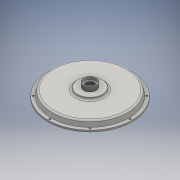
# Autodesk Inventor part: Flasque 1
Saved by Autodesk Inventor 2016 (Build 200138000, 138)
## iProperties
Created: 2015-11-14
Part Number: Flasque 1
Material: Générique
Document SubType Name: Modeling
Designer: Cyril
Density: 1 g/cm^3
Appearance: Par défaut
Author: Cyril
Autodesk Inventor part; units mm, degrees
ref_plane "YZ Plane" through (0, 0, 0) normal (1, 0, 0) x (0, 1, 0)
ref_plane "XZ Plane" through (0, 0, 0) normal (0, 1, 0) x (-1, 0, 0)
ref_plane "XY Plane" through (0, 0, 0) normal (0, 0, 1) x (1, 0, 0)
sketch "Esquisse1" plane through (0, 0, 0) normal (1, 0, 0) x (0, 1, 0)
  line L0 (0, 0) -> (0, 42.75) construction
  line L1 (102.5, -2.5) -> (106.5, -2.5)
  line L2 (106.5, -2.5) -> (106.5, 0)
  line L3 (106.5, 0) -> (115, 0)
  line L4 (115, 0) -> (115, 4.6)
  line L5 (115, 4.6) -> (106, 4.6)
  line L6 (106, 4.6) -> (103.0675, 15.5441)
  arc A0 (103.0675, 15.5441) -> (98.2379, 19.25) centre (98.2379, 14.25) ccw
  line L7 (98.2379, 19.25) -> (40, 19.25)
  line L8 (15, 39.25) -> (16.5, 39.25)
  line L9 (16.5, 39.25) -> (17.5, 38.25)
  line L10 (17.5, 38.25) -> (17.5, 27.25)
  line L11 (17.5, 27.25) -> (16.5, 27.25)
  line L12 (16.5, 27.25) -> (16.5, 25.25)
  line L13 (16.5, 25.25) -> (34, 25.25)
  line L14 (34, 25.25) -> (35, 24.25)
  arc A1 (35, 24.25) -> (40, 19.25) centre (40, 24.25) ccw
  line L15 (98.6398, 14.75) -> (34.5, 14.75)
  line L16 (102.3296, 6.7069) -> (100.5717, 13.2676)
  arc A2 (100.5717, 13.2676) -> (98.6398, 14.75) centre (98.6398, 12.75) ccw
  line L17 (102.5, -2.5) -> (102.5, 5.4128)
  arc A3 (102.5, 5.4128) -> (102.3296, 6.7069) centre (97.5, 5.4128) ccw
  line L18 (29.5, 9.75) -> (29.5, 8.25)
  arc A4 (34.5, 14.75) -> (29.5, 9.75) centre (34.5, 9.75) ccw
  line L19 (29.5, 8.25) -> (22, 8.25)
  line L20 (22, 8.25) -> (22, 20.25)
  line L21 (22, 20.25) -> (18.5, 20.25)
  line L22 (18.5, 20.25) -> (18.5, 21.25)
  line L23 (18.5, 21.25) -> (11.7, 26.95)
  line L24 (11.7, 26.95) -> (11.7, 32.25)
  line L25 (11.7, 32.25) -> (15, 32.25)
  line L26 (15, 32.25) -> (15, 39.25)
  line L27 (40, 24.25) -> (35, 24.25) construction
  dimension "d0" = 115
  dimension "d1" = 106.5
  dimension "d3" = 2.5
  dimension "d4" = 4.6
  dimension "d5" = 0.5
  dimension "d8" = 5
  dimension "d16" = 105
  dimension "d17" = 42.75
  dimension "d40" = 39.25
  dimension "d42" = 1
  dimension "d43" = 1
  dimension "d45" = 1
  dimension "d46" = 2
  dimension "d47" = 1
  dimension "d48" = 1
  dimension "d49" = 5
  dimension "d50" = 17.5
  dimension "d51" = 35
  dimension "d56" = 23.5
  dimension "d57" = 3
  dimension "d58" = 4.5
  dimension "d59" = 2
  dimension "d60" = 102.5
  dimension "d61" = 5
  dimension "d62" = 5
  dimension "d63" = 22
  dimension "d64" = 29.5
  dimension "d65" = 17
  dimension "d66" = 12
  dimension "d67" = 18.5
  dimension "d68" = 1
  dimension "d69" = 5.7
  dimension "d70" = 6.8
  dimension "d71" = 7
  dimension "d72" = 15
  constraints: 56 end point, 10 horizontal, 10 point on circle, 9 tangent, 8 vertical, 5 centre point, 5 perpendicular, 3 point on line, 1 parallel
  measures "d0" distance between parallel lines of L0 L4
  measures "d1" distance between parallel lines of L0 L2
  measures "d3" distance of L1.end L2.end
  measures "d4" distance of L3.end L4.end
  measures "d5" distance from line of L2 L5.end
  measures "d8" radius of A0
  measures "d16" angle of L5 L6
  measures "d17" distance of L0.start L0.end
  measures "d40" distance between parallel lines of L3 L8
  measures "d42" horizontal distance of L8.end L9.end
  measures "d43" horizontal distance of L8.end L9.end
  measures "d45" distance of L10.end L11.end
  measures "d46" distance of L11.end L12.end
  measures "d47" horizontal distance of L13.end L14.end
  measures "d48" horizontal distance of L13.end L14.end
  measures "d49" radius of A1
  measures "d50" distance between parallel lines of L0 L10
  measures "d51" distance from line of L0 L14.end
  measures "d56" distance from line of L7 L0.end
  measures "d57" distance between parallel lines of L16 L6
  measures "d58" distance between parallel lines of L7 L15
  measures "d59" radius of A2
  measures "d60" distance between parallel lines of L0 L17
  measures "d61" radius of A3
  measures "d62" radius of A4
  measures "d63" distance between parallel lines of L0 L20
  measures "d64" distance between parallel lines of L0 L18
  measures "d65" distance between parallel lines of L13 L19
  measures "d66" distance of L19.end L20.end
  measures "d67" distance between parallel lines of L0 L22
  measures "d68" distance of L21.end L22.end
  measures "d69" vertical distance of L22.end L23.end
  measures "d70" horizontal distance of L22.end L23.end
  measures "d71" distance of L25.end L8.start
  measures "d72" distance between parallel lines of L0 L26
revolve "Révolution1" add sketch "Esquisse1" angle 360 about axis through (0, 0, 0) along (0, 0, 1)
sketch "Esquisse2" plane through (0, 0, 4.6) normal (0, 0, 1) x (1, 0, 0)
  circle A0 centre (-110, 0) radius 2.65
  circle A1 centre (-77.7817, 77.7817) radius 2.65
  circle A2 centre (0, 110) radius 2.65
  circle A3 centre (77.7817, 77.7817) radius 2.65
  circle A4 centre (110, 0) radius 2.65
  circle A5 centre (77.7817, -77.7817) radius 2.65
  circle A6 centre (0, -110) radius 2.65
  circle A7 centre (-77.7817, -77.7817) radius 2.65
  line L0 (0, 0) -> (-110, 0) construction
  dimension "d19" = 5.3
  dimension "d22" = 360
  dimension "d24" = 220
  constraints: 8 centre point, 2 coincident, 2 end point, 1 horizontal, 22 other
  measures "d19" diameter of A0
  measures "d24" distance of A4.centre L0.end
extrude "Extrusion1" cut sketch "Esquisse2" against normal through all
thread "Filetage1" size "M35x1.5" class "6g" standard "ANSI Metric M Profile" full length
thread "Filetage2" size "M35x1.5" class "6g" standard "ANSI Metric M Profile" full length
